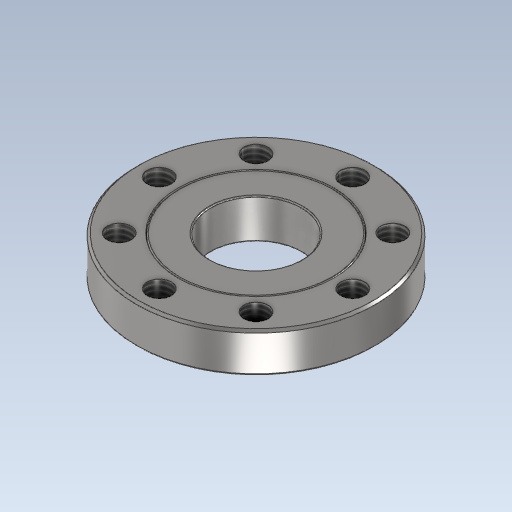
# Autodesk Inventor part: FreeHorn
Saved by Autodesk Inventor 2020 (Build 240168000, 168)
## iProperties
Part Number: FreeHorn
Material: アルミニウム 2014-T4
Document SubType Name: Modeling
Designer: Masato Kubotera
Density: 2.8 g/cm^3
Appearance: 半つや出し
Catalog Web Link: https://kondo-robot.com/product/02137
Description: ReadyMade
Mass: 2.61178 g
Surface Area: 10.9898 cm^2
Volume: 0.93278 cm^3
Author: MasatoKubotera
Autodesk Inventor part; units mm, degrees
ref_plane "YZ Plane" through (0, 0, 0) normal (1, 0, 0) x (0, 1, 0)
ref_plane "XZ Plane" through (0, 0, 0) normal (0, 1, 0) x (-1, 0, 0)
ref_plane "XY Plane" through (0, 0, 0) normal (0, 0, 1) x (1, 0, 0)
sketch "スケッチ1" plane through (0, 0, 0) normal (0, 1, 0) x (-1, 0, 0)
  line L0 (-6.2, 0) -> (-10.5, 0)
  line L1 (-10.5, 0) -> (-10.5, 3.5)
  line L2 (-10.5, 3.5) -> (-6.85, 3.5)
  line L3 (-6.85, 3.5) -> (-6.85, 2.7)
  line L4 (-6.85, 2.7) -> (-6.8, 2.7)
  line L5 (-6.8, 3.4) -> (-6.8, 2.7)
  line L6 (-6, 0.2) -> (-6, 0.1)
  line L7 (-5.9, 0) -> (-4.1, 0)
  line L8 (-4, 0.1) -> (-4, 3.4)
  line L9 (-4.1, 3.5) -> (-6.7, 3.5)
  line L10 (0, -0.729) -> (0, 4.229) projected
  line L11 (-6, 0.2) -> (-6.2, 0)
  arc A0 (-6.7, 3.5) -> (-6.8, 3.4) centre (-6.7, 3.4) ccw
  arc A1 (-4, 3.4) -> (-4.1, 3.5) centre (-4.1, 3.4) ccw
  arc A2 (-4.1, 0) -> (-4, 0.1) centre (-4.1, 0.1) ccw
  arc A3 (-6, 0.1) -> (-5.9, 0) centre (-5.9, 0.1) ccw
  line L12 (2.1, 0) -> (-12.6, 0) projected
  point P0 (0, 0)
  point P1 (-6.8, 3.5)
  point P2 (-6, 0)
  point P3 (-4, 0)
  point P4 (-4, 3.5)
  dimension "d0" = 8
  dimension "d1" = 21
  dimension "d2" = 0.8
  dimension "d3" = 0.1
  dimension "d4" = 13.7
  dimension "d5" = 13.6
  dimension "d6" = 0.2
  dimension "d7" = 0.2
  dimension "d8" = 12
  dimension "d9" = 3.5
  constraints: 22 end point, 12 point on line, 8 point on circle, 8 tangent, 7 perpendicular, 4 centre point, 3 equal radius, 1 collinear, 1 horizontal
  measures "d0" diameter of L8 L10
  measures "d1" diameter of L1 L10
  measures "d2" distance of L2.end L3.end
  measures "d3" radius of A0
  measures "d4" diameter of L3 L10
  measures "d5" diameter of L5 L10
  measures "d6" horizontal distance of L0.start L6.start
  measures "d7" horizontal distance of L0.start L6.start
  measures "d8" diameter of L6 L10
  measures "d9" distance of L0.end L1.end
revolve "回転1" add sketch "スケッチ1" angle 360 about axis through (0, 0, -10) along (0, 0, 1) contours L0 L1 L2 L3 L4 L5 A0 L9 A1 L8 A2 L7 A3 L6 L11
sketch "スケッチ2" plane through (0, 0, 3.5) normal (0, 0, 1) x (1, 0, 0)
  line L0 (-14.7, 0) -> (14.7, 0) projected
  point P0 (0, 0)
  point P1 (-8.5, 0)
  dimension "d12" = 8.5
  constraints: 1 point on line
  measures "d12" distance of point (0, 0) point (-8.5, 0)
hole "穴1" at (-8.5, 0, 3.5) direction (0, 0, -1) diameter 2.1129 end through all thread size "M2.6x0.45" class "6H" standard "ISO Metric profile"
pattern_circular "円形状パターン1" count 8 over 360 about axis through (0, 0, -10) along (0, 0, 1) of "穴1"
chamfer "面取り1" distance 0.2 angle 45 2 edges at (-10.5, 0, 3.5) (-10.5, 0, 0)
